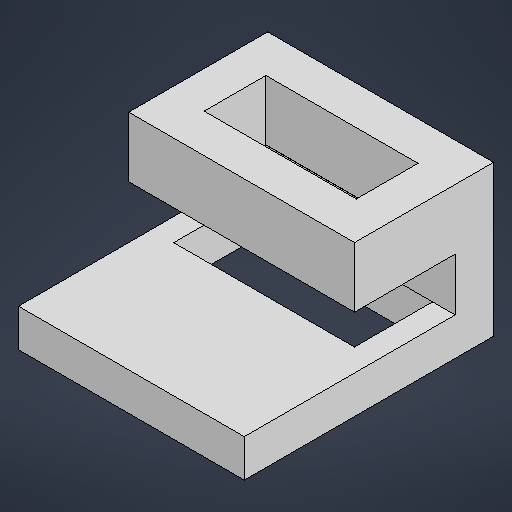
# Autodesk Inventor part: LRA_case2
Saved by Autodesk Inventor 2026 (Build 300175050, 175E)
## iProperties
Created: 2025-09-05
Part Number: LRA_case2
Material: 一般
Document SubType Name: Modeling
Designer: ka0n7
Density: 1 g/cm^3
Appearance: 既定
Author: ka0n7
Autodesk Inventor part; units mm, degrees
ref_plane "YZ Plane" through (0, 0, 0) normal (1, 0, 0) x (0, 1, 0)
ref_plane "XZ Plane" through (0, 0, 0) normal (0, 1, 0) x (-1, 0, 0)
ref_plane "XY Plane" through (0, 0, 0) normal (0, 0, 1) x (1, 0, 0)
sketch "スケッチ1" plane through (0, 0, 0) normal (0, 1, 0) x (-1, 0, 0)
  line L0 (5.05, 2.05) -> (-5.05, 2.05)
  line L1 (-5.05, 2.05) -> (-5.05, -2.05)
  line L2 (-5.05, -2.05) -> (5.05, -2.05)
  line L3 (5.05, -2.05) -> (5.05, 2.05)
  line L4 (5.05, 2.05) -> (-5.05, -2.05) construction
  line L5 (-5.05, 2.05) -> (5.05, -2.05) construction
  line L6 (7.5, 4.6151) -> (-7.5, 4.6151)
  line L7 (-7.5, 4.6151) -> (-7.5, -4.6151)
  line L8 (-7.5, -4.6151) -> (7.5, -4.6151)
  line L9 (7.5, -4.6151) -> (7.5, 4.6151)
  line L10 (7.5, 4.6151) -> (-7.5, -4.6151) construction
  line L11 (-7.5, 4.6151) -> (7.5, -4.6151) construction
  point P0 (0, 0)
  dimension "d0" = 10.1
  dimension "d1" = 4.1
  dimension "d2" = 15
  constraints: 24 end point, 4 midpoint, 4 parallel, 2 horizontal, 2 perpendicular
  measures "d0" distance of L2.end L1.end
  measures "d1" distance of L2.end L0.start
  measures "d2" distance of L8.end L7.end
extrude "押し出し1" add sketch "スケッチ1" along normal blind 4
sketch "スケッチ2" plane through (0, 0, 0) normal (0, -1, 0) x (1, 0, 0)
  line L0 (7.5, 4.6151) -> (7.5, -4.6151) projected
  line L1 (-7.5, -4.6151) -> (7.5, -4.6151)
  line L2 (7.5, -4.6151) -> (7.5, -2.0651)
  line L3 (7.5, -2.0651) -> (-7.5, -2.0651)
  line L4 (-7.5, -2.0651) -> (-7.5, -4.6151)
  point P0 (0, 0)
  dimension "d5" = 2.55
  constraints: 8 end point, 2 parallel, 1 horizontal, 1 perpendicular, 1 point on line
  measures "d5" distance between parallel lines of L3 L1
extrude "押し出し2" add sketch "スケッチ2" along normal blind 6
sketch "スケッチ3" plane through (-7.5, 0, -2.0651) normal (0, 0, 1) x (1, 0, 0)
  line L0 (15, -6) -> (0, -6) projected
  line L1 (15, -6) -> (15, 4) projected
  line L2 (0, -6) -> (15, -6)
  line L3 (15, -6) -> (15, -3.5)
  line L4 (15, -3.5) -> (0, -3.5)
  line L5 (0, -3.5) -> (0, -6)
  point P0 (7.5, 0)
  dimension "d8" = 2.5
  constraints: 8 end point, 2 parallel, 1 horizontal, 1 perpendicular, 1 point on line
  measures "d8" distance between parallel lines of L0 L4
extrude "押し出し3" add sketch "スケッチ3" along normal blind 14
sketch "スケッチ4" plane through (-7.5, -3.5, -2.0651) normal (0, 1, 0) x (1, 0, 0)
  line L0 (1.5, 1.0597) -> (13.5, 1.0597)
  line L1 (13.5, 1.0597) -> (13.5, -5.1899)
  line L2 (13.5, -5.1899) -> (1.5, -5.1899)
  line L3 (1.5, -5.1899) -> (1.5, 1.0597)
  line L4 (1.5, 1.0597) -> (13.5, -5.1899) construction
  line L5 (13.5, 1.0597) -> (1.5, -5.1899) construction
  line L6 (1.5, -0.0039) -> (13.5, 0)
  line L7 (0, 0) -> (15, 0) projected
  point P0 (7.5, -2.0651)
  dimension "d11" = 12
  constraints: 14 end point, 3 point on line, 2 midpoint, 2 parallel, 1 horizontal, 1 perpendicular
  measures "d11" distance of L1.end L2.end
extrude "押し出し4" cut sketch "スケッチ4" against normal blind 10 contours L1 L2 L3 L6
